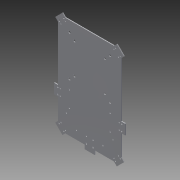
# Autodesk Inventor part: Main Plate
Saved by Autodesk Inventor 2013 (Build 170138000, 138)
## iProperties
Created: 2014-05-12
Part Number: Main Plate
Material: アルミニウム 6061
Document SubType Name: Modeling
Designer: andou
Density: 2.71 g/cm^3
Mass: 218.036 g
Surface Area: 829.556 cm^2
Volume: 80.4562 cm^3
Author: andou
Autodesk Inventor part; units mm, degrees
ref_plane "YZ Plane" through (0, 0, 0) normal (1, 0, 0) x (0, 1, 0)
ref_plane "XZ Plane" through (0, 0, 0) normal (0, 1, 0) x (-1, 0, 0)
ref_plane "XY Plane" through (0, 0, 0) normal (0, 0, 1) x (1, 0, 0)
sketch "スケッチ1" plane through (0, 0, 0) normal (0, 1, 0) x (-1, 0, 0)
  line L0 (-84.7487, 117.8934) -> (-67.0711, 135.5711)
  line L1 (-67.0711, 135.5711) -> (-60, 128.5)
  line L2 (-60, 128.5) -> (0, 128.5)
  line L3 (-84.7487, 117.8934) -> (-77.6777, 110.8223)
  line L4 (-77.6777, 110.8223) -> (-77.6777, -24.1777)
  line L5 (-77.6777, -24.1777) -> (-87.6777, -24.1777)
  line L6 (-87.6777, -24.1777) -> (-87.6777, -49.1777)
  line L7 (-87.6777, -49.1777) -> (-77.6777, -49.1777)
  line L8 (-77.6777, -49.1777) -> (-77.6777, -100.8223)
  line L9 (-77.6777, -100.8223) -> (-84.7487, -107.8934)
  line L10 (-84.7487, -107.8934) -> (-67.0711, -125.5711)
  line L11 (-67.0711, -125.5711) -> (-60, -118.5)
  line L12 (-60, -118.5) -> (-12.5, -118.5)
  line L13 (-12.5, -118.5) -> (-12.5, -128.5)
  line L14 (-12.5, -128.5) -> (0, -128.5)
  line L15 (0, -128.5) -> (0, 128.5)
  line L16 (84.7487, 117.8934) -> (67.0711, 135.5711)
  line L17 (67.0711, 135.5711) -> (60, 128.5)
  line L18 (60, 128.5) -> (0, 128.5)
  line L19 (84.7487, 117.8934) -> (77.6777, 110.8223)
  line L20 (77.6777, 110.8223) -> (77.6777, -24.1777)
  line L21 (77.6777, -24.1777) -> (87.6777, -24.1777)
  line L22 (87.6777, -24.1777) -> (87.6777, -49.1777)
  line L23 (87.6777, -49.1777) -> (77.6777, -49.1777)
  line L24 (77.6777, -49.1777) -> (77.6777, -100.8223)
  line L25 (77.6777, -100.8223) -> (84.7487, -107.8934)
  line L26 (84.7487, -107.8934) -> (67.0711, -125.5711)
  line L27 (67.0711, -125.5711) -> (60, -118.5)
  line L28 (60, -118.5) -> (12.5, -118.5)
  line L29 (12.5, -118.5) -> (12.5, -128.5)
  line L30 (12.5, -128.5) -> (0, -128.5)
  point P0 (0, 0)
  dimension "d0" = 135
  dimension "d2" = 135
  dimension "d4" = 10
  dimension "d6" = 128.5
  dimension "d8" = 25
  dimension "d9" = 257
  dimension "d10" = 12.5
  dimension "d12" = 60
  dimension "d13" = 0
  dimension "d40" = 10
  constraints: 62 end point, 14 symmetric about line, 12 perpendicular, 7 equal length, 2 parallel, 1 horizontal
  measures "d0" distance of L3.end L4.end
  measures "d2" angle of L2 L1
  measures "d4" distance of L0.end L1.end
  measures "d6" distance of L2.end point (0, 0)
  measures "d8" distance of L5.end L6.end
  measures "d9" distance of L14.end L2.end
  measures "d10" distance of L13.end L14.end
  measures "d12" distance of L1.end L2.end
  measures "d13" distance from line of point (0, 0) L15
  measures "d40" distance of L8.end L9.end
extrude "押し出し1" add sketch "スケッチ1" along normal blind 2
sketch "スケッチ2" plane through (0, 2, 0) normal (0, 1, 0) x (1, 0, 0)
  line L0 (12.5, 128.5) -> (-12.5, 128.5) projected
  line L1 (-67.0711, 125.5711) -> (-84.7487, 107.8934) projected
  line L2 (-84.7487, 107.8934) -> (-77.6777, 100.8223) projected
  line L3 (-87.6777, 49.1777) -> (-87.6777, 24.1777) projected
  line L4 (-87.6777, 24.1777) -> (-77.6777, 24.1777) projected
  line L5 (-84.7487, -117.8934) -> (-67.0711, -135.5711) projected
  line L6 (-67.0711, -135.5711) -> (-60, -128.5) projected
  line L7 (-60, -128.5) -> (60, -128.5) projected
  circle A0 centre (-59.6464, 111.7825) radius 1.6
  circle A1 centre (-70.9602, 100.4688) radius 1.6
  circle A2 centre (-8, 98.5) radius 1.6
  circle A3 centre (-72.6777, 44.6777) radius 1.6
  circle A4 centre (-72.6777, 28.6777) radius 1.6
  circle A5 centre (-70.9602, -110.4688) radius 1.6
  circle A6 centre (-59.6464, -121.7825) radius 1.6
  line L8 (0, 128.5) -> (0, -128.5)
  circle A7 centre (59.6464, 111.7825) radius 1.6
  circle A8 centre (70.9602, 100.4688) radius 1.6
  circle A9 centre (8, 98.5) radius 1.6
  circle A10 centre (72.6777, 44.6777) radius 1.6
  circle A11 centre (72.6777, 28.6777) radius 1.6
  circle A12 centre (70.9602, -110.4688) radius 1.6
  circle A13 centre (59.6464, -121.7825) radius 1.6
  point P0 (0, 0)
  dimension "d16" = 3.2
  dimension "d17" = 30
  dimension "d18" = 8
  dimension "d21" = 15
  dimension "d22" = 15
  dimension "d23" = 16
  dimension "d24" = 4.5
  dimension "d25" = 15
  dimension "d26" = 15
  dimension "d27" = 16
  dimension "d28" = 4.5
  dimension "d29" = 15
  dimension "d30" = 15
  dimension "d31" = 16
  dimension "d32" = 4.5
  constraints: 14 centre point, 7 symmetric about line, 6 equal radius, 2 end point, 2 midpoint, 7 other
  measures "d16" diameter of A2
  measures "d17" distance from line of L0 A2.centre
  measures "d18" distance from line of L8 A2.centre
  measures "d21" distance from line of L1 A0.centre
  measures "d22" distance from line of L1 A1.centre
  measures "d23" distance of A0.centre A1.centre
  measures "d24" distance from line of L2 A1.centre
  measures "d25" distance from line of L3 A3.centre
  measures "d26" distance from line of L3 A4.centre
  measures "d27" distance of A3.centre A4.centre
  measures "d28" distance from line of A4.centre L4
  measures "d29" distance from line of A5.centre L5
  measures "d30" distance from line of A6.centre L5
  measures "d31" distance of A5.centre A6.centre
  measures "d32" distance from line of L6 A6.centre
hole "穴1" at (-59.6464, 2, -111.7825) at (-70.9602, 2, -100.4688) at (-72.6777, 2, -44.6777) at (-72.6777, 2, -28.6777) at (-8, 2, -98.5) at (8, 2, -98.5) at (59.6464, 2, -111.7825) at (70.9602, 2, -100.4688) at (-70.9602, 2, 110.4688) at (-59.6464, 2, 121.7825) at (59.6464, 2, 121.7825) at (70.9602, 2, 110.4688) at (72.6777, 2, -28.6777) at (72.6777, 2, -44.6777) direction (0, -1, 0) diameter 3.5 end through all
sketch "スケッチ3" plane through (0, 0, 0) normal (0, -1, 0) x (1, 0, 0)
  line L0 (-60, 128.5) -> (60, 128.5) projected
  circle A0 centre (-37.5, 90) radius 2.5
  circle A1 centre (-50, 102.5) radius 2.5
  circle A2 centre (-37.5, 15) radius 2.5
  circle A3 centre (-50, 2.5) radius 2.5
  line L1 (0, 0) -> (0, 128.5)
  circle A4 centre (37.5, 90) radius 2.5
  circle A5 centre (50, 2.5) radius 2.5
  circle A6 centre (37.5, 90) radius 2.5
  circle A7 centre (50, 102.5) radius 2.5
  circle A8 centre (37.5, 15) radius 2.5
  circle A9 centre (50, 2.5) radius 2.5
  dimension "d41" = 5
  dimension "d44" = 100
  dimension "d45" = 75
  dimension "d46" = 12.5
  dimension "d47" = 37.5
  dimension "d48" = 50
  dimension "d49" = 37.5
  dimension "d50" = 50
  dimension "d51" = 15
  constraints: 10 centre point, 8 symmetric about line, 3 equal radius, 2 end point, 1 midpoint, 6 other
  measures "d41" diameter of A1
  measures "d44" distance of A1.centre A3.centre
  measures "d45" distance of A0.centre A2.centre
  measures "d46" horizontal distance of A1.centre A0.centre
  measures "d47" horizontal distance of A2.centre L1.start
  measures "d48" horizontal distance of L1.start A3.centre
  measures "d49" horizontal distance of L1.start A0.centre
  measures "d50" horizontal distance of L1.start A1.centre
  measures "d51" vertical distance of A2.centre L1.start
hole "穴2" at (-37.5, 0, 90) at (-50, 0, 102.5) at (-37.5, 0, 15) at (-50, 0, 2.5) at (37.5, 0, 15) at (50, 0, 2.5) at (37.5, 0, 90) at (50, 0, 102.5) direction (0, 1, 0) diameter 5.5 end through all
sketch "スケッチ5" plane through (0, 2, 0) normal (0, 1, 0) x (1, 0, 0)
  line L0 (77.6777, 100.8223) -> (84.7487, 107.8934) projected
  line L1 (84.7487, 107.8934) -> (67.0711, 125.5711) projected
  line L2 (-67.0711, 125.5711) -> (-84.7487, 107.8934) projected
  line L3 (-84.7487, 107.8934) -> (-77.6777, 100.8223) projected
  circle A0 centre (-57.1716, 73.2452) radius 1.5
  circle A1 centre (-32.4228, 97.9939) radius 1.5
  circle A2 centre (32.4228, 97.9939) radius 1.5
  circle A3 centre (57.1716, 73.2452) radius 1.5
  line L4 (-32.4228, 97.9939) -> (-57.1716, 73.2452)
  line L5 (32.4228, 97.9939) -> (57.1716, 73.2452)
  circle A4 centre (-75.2028, 104.7114) radius 1.5
  circle A5 centre (-63.8891, 116.0251) radius 1.5
  circle A6 centre (37.5, -90) radius 2.75 projected
  circle A7 centre (37.5, -15) radius 2.75 projected
  circle A8 centre (-37.5, -15) radius 2.75 projected
  circle A9 centre (-37.5, -90) radius 2.75 projected
  circle A10 centre (-50, -102.5) radius 2.75 projected
  circle A11 centre (-50, -2.5) radius 2.75 projected
  circle A12 centre (50, -2.5) radius 2.75 projected
  circle A13 centre (50, -102.5) radius 2.75 projected
  circle A14 centre (72.6777, 28.6777) radius 1.75 projected
  circle A15 centre (59.6464, -121.7825) radius 1.75 projected
  circle A16 centre (-70.9602, -110.4688) radius 1.75 projected
  circle A17 centre (59.6464, 111.7825) radius 1.75 projected
  circle A18 centre (-8, 98.5) radius 1.75 projected
  circle A19 centre (-72.6777, 44.6777) radius 1.75 projected
  circle A20 centre (-59.6464, 111.7825) radius 1.75 projected
  circle A21 centre (-70.9602, 100.4688) radius 1.75 projected
  circle A22 centre (-72.6777, 28.6777) radius 1.75 projected
  circle A23 centre (8, 98.5) radius 1.75 projected
  circle A24 centre (70.9602, 100.4688) radius 1.75 projected
  circle A25 centre (-59.6464, -121.7825) radius 1.75 projected
  circle A26 centre (70.9602, -110.4688) radius 1.75 projected
  circle A27 centre (72.6777, 44.6777) radius 1.75 projected
  line L6 (84.7487, -117.8934) -> (77.6777, -110.8223) projected
  line L7 (77.6777, -110.8223) -> (77.6777, 24.1777) projected
  line L8 (77.6777, 24.1777) -> (87.6777, 24.1777) projected
  line L9 (87.6777, 24.1777) -> (87.6777, 49.1777) projected
  line L10 (87.6777, 49.1777) -> (77.6777, 49.1777) projected
  line L11 (77.6777, 49.1777) -> (77.6777, 100.8223) projected
  line L12 (77.6777, 100.8223) -> (84.7487, 107.8934) projected
  line L13 (84.7487, 107.8934) -> (67.0711, 125.5711) projected
  line L14 (67.0711, 125.5711) -> (60, 118.5) projected
  line L15 (60, 118.5) -> (12.5, 118.5) projected
  line L16 (12.5, 118.5) -> (12.5, 128.5) projected
  line L17 (12.5, 128.5) -> (-12.5, 128.5) projected
  line L18 (-12.5, 128.5) -> (-12.5, 118.5) projected
  line L19 (-12.5, 118.5) -> (-60, 118.5) projected
  line L20 (-60, 118.5) -> (-67.0711, 125.5711) projected
  line L21 (-67.0711, 125.5711) -> (-84.7487, 107.8934) projected
  line L22 (-84.7487, 107.8934) -> (-77.6777, 100.8223) projected
  line L23 (-77.6777, 100.8223) -> (-77.6777, 49.1777) projected
  line L24 (-77.6777, 49.1777) -> (-87.6777, 49.1777) projected
  line L25 (-87.6777, 49.1777) -> (-87.6777, 24.1777) projected
  line L26 (-87.6777, 24.1777) -> (-77.6777, 24.1777) projected
  line L27 (-77.6777, 24.1777) -> (-77.6777, -110.8223) projected
  line L28 (-77.6777, -110.8223) -> (-84.7487, -117.8934) projected
  line L29 (-84.7487, -117.8934) -> (-67.0711, -135.5711) projected
  line L30 (-67.0711, -135.5711) -> (-60, -128.5) projected
  line L31 (-60, -128.5) -> (60, -128.5) projected
  line L32 (60, -128.5) -> (67.0711, -135.5711) projected
  line L33 (67.0711, -135.5711) -> (84.7487, -117.8934) projected
  line L34 (-75.2028, 104.7114) -> (-63.8891, 116.0251)
  circle A28 centre (63.8891, 116.0251) radius 1.5
  circle A29 centre (75.2028, 104.7114) radius 1.5
  line L35 (63.8891, 116.0251) -> (75.2028, 104.7114)
  point P0 (0, 0)
  dimension "d64" = 3
  dimension "d65" = 35
  dimension "d68" = 5
  dimension "d69" = 5
  dimension "d77" = 16
  dimension "d80" = 4.5
  dimension "d82" = 4.5
  dimension "d83" = 16
  dimension "d129" = 6
  dimension "d130" = 35
  dimension "d131" = 6
  dimension "d132" = 35
  constraints: 8 centre point, 8 end point, 7 equal radius, 3 perpendicular, 2 parallel, 1 coincident
  measures "d64" diameter of A1
  measures "d65" distance of A1.centre L4.end
  measures "d68" distance from line of L4.end L3
  measures "d69" distance from line of L0 L5.end
  measures "d77" distance of L34.end L34.start
  measures "d80" distance from line of L3 L34.start
  measures "d82" distance from line of L0 L35.end
  measures "d83" distance of L35.start L35.end
  measures "d129" distance from line of L34 A20.centre
  measures "d130" distance between parallel lines of L4 L34
  measures "d131" distance from line of L35 A24.centre
  measures "d132" distance between parallel lines of L35 L5
hole "穴4" at (-75.2028, 2, -104.7114) at (-63.8891, 2, -116.0251) at (-57.1716, 2, -73.2452) at (-32.4228, 2, -97.9939) at (32.4228, 2, -97.9939) at (57.1716, 2, -73.2452) at (75.2028, 2, -104.7114) at (63.8891, 2, -116.0251) direction (0, -1, 0) diameter 3.5 end through all
sketch "スケッチ6" plane through (0, 2, 0) normal (0, 1, 0) x (1, 0, 0)
  circle A0 centre (-50, 60) radius 1.75
  circle A1 centre (-50, 20) radius 1.75
  circle A2 centre (50, 60) radius 1.75
  circle A3 centre (50, 20) radius 1.75
  point P0 (0, 0)
  dimension "d91" = 100
  dimension "d93" = 100
  dimension "d94" = 40
  dimension "d95" = 40
  dimension "d96" = 3.5
  dimension "d97" = 60
  dimension "d98" = 60
  dimension "d99" = 50
  dimension "d100" = 50
  constraints: 4 centre point, 3 equal radius
  measures "d91" distance of A2.centre A0.centre
  measures "d93" distance of A3.centre A1.centre
  measures "d94" distance of A0.centre A1.centre
  measures "d95" distance of A2.centre A3.centre
  measures "d96" diameter of A2
  measures "d97" vertical distance of point (0, 0) A0.centre
  measures "d98" vertical distance of point (0, 0) A2.centre
  measures "d99" horizontal distance of point (0, 0) A3.centre
  measures "d100" horizontal distance of point (0, 0) A0.centre
hole "穴5" at (-50, 2, -60) at (-50, 2, -20) at (50, 2, -60) at (50, 2, -20) direction (0, -1, 0) diameter 3.5 end through all
sketch "スケッチ7" plane through (0, 2, 0) normal (0, 1, 0) x (1, 0, 0)
  circle A0 centre (50, 60) radius 1.75 projected
  circle A1 centre (-50, 60) radius 1.75 projected
  circle A2 centre (-50, 20) radius 1.75 projected
  circle A3 centre (50, 20) radius 1.75 projected
  circle A4 centre (75.2028, 104.7114) radius 1.75 projected
  circle A5 centre (32.4228, 97.9939) radius 1.75 projected
  circle A6 centre (-57.1716, 73.2452) radius 1.75 projected
  circle A7 centre (-75.2028, 104.7114) radius 1.75 projected
  circle A8 centre (-63.8891, 116.0251) radius 1.75 projected
  circle A9 centre (-32.4228, 97.9939) radius 1.75 projected
  circle A10 centre (57.1716, 73.2452) radius 1.75 projected
  circle A11 centre (63.8891, 116.0251) radius 1.75 projected
  circle A12 centre (37.5, -90) radius 2.75 projected
  circle A13 centre (37.5, -15) radius 2.75 projected
  circle A14 centre (-37.5, -15) radius 2.75 projected
  circle A15 centre (-37.5, -90) radius 2.75 projected
  circle A16 centre (-50, -102.5) radius 2.75 projected
  circle A17 centre (-50, -2.5) radius 2.75 projected
  circle A18 centre (50, -2.5) radius 2.75 projected
  circle A19 centre (50, -102.5) radius 2.75 projected
  circle A20 centre (72.6777, 28.6777) radius 1.75 projected
  circle A21 centre (59.6464, -121.7825) radius 1.75 projected
  circle A22 centre (-70.9602, -110.4688) radius 1.75 projected
  circle A23 centre (59.6464, 111.7825) radius 1.75 projected
  circle A24 centre (-8, 98.5) radius 1.75 projected
  circle A25 centre (-72.6777, 44.6777) radius 1.75 projected
  circle A26 centre (-59.6464, 111.7825) radius 1.75 projected
  circle A27 centre (-70.9602, 100.4688) radius 1.75 projected
  circle A28 centre (-72.6777, 28.6777) radius 1.75 projected
  circle A29 centre (8, 98.5) radius 1.75 projected
  circle A30 centre (70.9602, 100.4688) radius 1.75 projected
  circle A31 centre (-59.6464, -121.7825) radius 1.75 projected
  circle A32 centre (70.9602, -110.4688) radius 1.75 projected
  circle A33 centre (72.6777, 44.6777) radius 1.75 projected
  line L0 (84.7487, -117.8934) -> (77.6777, -110.8223) projected
  line L1 (77.6777, -110.8223) -> (77.6777, 24.1777) projected
  line L2 (77.6777, 24.1777) -> (87.6777, 24.1777) projected
  line L3 (87.6777, 24.1777) -> (87.6777, 49.1777) projected
  line L4 (87.6777, 49.1777) -> (77.6777, 49.1777) projected
  line L5 (77.6777, 49.1777) -> (77.6777, 100.8223) projected
  line L6 (77.6777, 100.8223) -> (84.7487, 107.8934) projected
  line L7 (84.7487, 107.8934) -> (67.0711, 125.5711) projected
  line L8 (67.0711, 125.5711) -> (60, 118.5) projected
  line L9 (60, 118.5) -> (12.5, 118.5) projected
  line L10 (12.5, 118.5) -> (12.5, 128.5) projected
  line L11 (12.5, 128.5) -> (-12.5, 128.5) projected
  line L12 (-12.5, 128.5) -> (-12.5, 118.5) projected
  line L13 (-12.5, 118.5) -> (-60, 118.5) projected
  line L14 (-60, 118.5) -> (-67.0711, 125.5711) projected
  line L15 (-67.0711, 125.5711) -> (-84.7487, 107.8934) projected
  line L16 (-84.7487, 107.8934) -> (-77.6777, 100.8223) projected
  line L17 (-77.6777, 100.8223) -> (-77.6777, 49.1777) projected
  line L18 (-77.6777, 49.1777) -> (-87.6777, 49.1777) projected
  line L19 (-87.6777, 49.1777) -> (-87.6777, 24.1777) projected
  line L20 (-87.6777, 24.1777) -> (-77.6777, 24.1777) projected
  line L21 (-77.6777, 24.1777) -> (-77.6777, -110.8223) projected
  line L22 (-77.6777, -110.8223) -> (-84.7487, -117.8934) projected
  line L23 (-84.7487, -117.8934) -> (-67.0711, -135.5711) projected
  line L24 (-67.0711, -135.5711) -> (-60, -128.5) projected
  line L25 (-60, -128.5) -> (60, -128.5) projected
  line L26 (60, -128.5) -> (67.0711, -135.5711) projected
  line L27 (67.0711, -135.5711) -> (84.7487, -117.8934) projected
  line L28 (-30, 60) -> (0, 47.5736)
  line L29 (0, 47.5736) -> (30, 60)
  line L30 (30, 60) -> (-30, 60)
  line L31 (-50, 50) -> (-50, 30)
  line L32 (-50, 30) -> (-12.6795, 40)
  line L33 (-12.6795, 40) -> (-50, 50)
  line L34 (-38.2518, -17.6489) -> (-36.0663, -17.3467)
  line L35 (-38.2518, -17.6452) -> (-38.2518, -17.6489)
  line L36 (-30, 0) -> (30, 0)
  line L37 (30, 0) -> (0, -30)
  line L38 (0, -30) -> (-30, 0)
  line L39 (0, 60) -> (0, 20)
  line L40 (-50, 40) -> (50, 40)
  line L41 (-50, -2.5) -> (0, -52.5)
  line L42 (50, -2.5) -> (0, -52.5)
  line L43 (-52.5, -82.5) -> (-52.5, -22.5)
  line L44 (-52.5, -22.5) -> (-22.5, -52.5)
  line L45 (-22.5, -52.5) -> (-52.5, -82.5)
  line L46 (30, -105) -> (-30, -105)
  line L47 (-30, -105) -> (0, -75)
  line L48 (0, -75) -> (30, -105)
  line L49 (52.5, -22.5) -> (52.5, -82.5)
  line L50 (52.5, -82.5) -> (22.5, -52.5)
  line L51 (22.5, -52.5) -> (52.5, -22.5)
  line L52 (-30, 20) -> (0, 32.4264)
  line L53 (0, 32.4264) -> (30, 20)
  line L54 (30, 20) -> (-30, 20)
  line L55 (50, 50) -> (50, 30)
  line L56 (50, 30) -> (12.6795, 40)
  line L57 (12.6795, 40) -> (50, 50)
  point P0 (0, 0)
  dimension "d109" = 135
  dimension "d110" = 60
  dimension "d112" = 20
  dimension "d113" = 0
  dimension "d114" = 0
  dimension "d115" = 20
  dimension "d116" = 10
  dimension "d117" = 30
  dimension "d119" = 60
  dimension "d120" = 20
  dimension "d121" = 90
  dimension "d122" = 0
  dimension "d125" = 360
  constraints: 60 end point, 7 perpendicular, 6 symmetric about line, 3 equal length, 2 midpoint, 2 point on circle, 1 parallel, 25 other
  measures "d109" angle of L29 L28
  measures "d110" distance of L29.end L28.start
  measures "d112" distance of A0.centre L29.end
  measures "d113" distance from line of A0.centre L30
  measures "d114" distance from line of A2.centre L31
  measures "d115" distance of L31.start L31.end
  measures "d116" distance of A1.centre L31.start
  measures "d117" angle of L33 L32
  measures "d119" distance of L36.start L36.end
  measures "d120" horizontal distance of L42.start L36.end
  measures "d121" angle of L37 L38
  measures "d122" distance from line of point (0, 0) L36
extrude "押し出し2" [suppressed]
sketch "スケッチ9" plane through (0, 0, 0) normal (0, -1, 0) x (1, 0, 0)
  circle A0 centre (-70.9602, 110.4688) radius 1.75 projected
  circle A1 centre (-8, -98.5) radius 1.75 projected
  circle A2 centre (-72.6777, -44.6777) radius 1.75 projected
  circle A3 centre (-59.6464, 121.7825) radius 1.75 projected
  line L0 (-60, 128.5) -> (60, 128.5) projected
  line L1 (-67.0711, 135.5711) -> (-60, 128.5) projected
  line L2 (-77.6777, 110.8223) -> (-84.7487, 117.8934) projected
  line L3 (-87.6777, -49.1777) -> (-87.6777, -24.1777) projected
  line L4 (-77.6777, -49.1777) -> (-87.6777, -49.1777) projected
  line L5 (-12.5, -128.5) -> (-12.5, -118.5) projected
  line L6 (12.5, -128.5) -> (-12.5, -128.5) projected
  line L7 (77.6777, 110.8223) -> (77.6777, -24.1777) projected
  circle A4 centre (-78.6777, -28.6777) radius 2
  circle A5 centre (-78.6777, -44.6777) radius 2
  circle A6 centre (-63.8891, 126.0251) radius 2
  circle A7 centre (-75.2028, 114.7114) radius 2
  line L8 (-78.6777, -44.6777) -> (-78.6777, -28.6777)
  line L9 (-75.2028, 114.7114) -> (-63.8891, 126.0251)
  line L10 (0, 128.5) -> (0, -128.5)
  circle A8 centre (-8, -114.5) radius 2
  circle A9 centre (78.6777, -28.6777) radius 2
  circle A10 centre (78.6777, -44.6777) radius 2
  circle A11 centre (63.8891, 126.0251) radius 2
  circle A12 centre (75.2028, 114.7114) radius 2
  circle A13 centre (8, -114.5) radius 2
  point P0 (0, 0)
  dimension "d133" = 4
  dimension "d135" = 6
  dimension "d136" = 4.5
  dimension "d137" = 16
  dimension "d142" = 4.5
  dimension "d143" = 4.5
  dimension "d144" = 6
  dimension "d145" = 6
  dimension "d146" = 16
  dimension "d147" = 4.5
  constraints: 10 centre point, 6 end point, 5 symmetric about line, 4 equal radius, 2 midpoint, 2 parallel, 5 other
  measures "d133" diameter of A6
  measures "d135" distance from line of A2.centre L8
  measures "d136" distance from line of L4 L8.start
  measures "d137" distance of L8.start L8.end
  measures "d142" distance from line of L9.start L2
  measures "d143" distance from line of L1 L9.end
  measures "d144" distance of L9.end A3.centre
  measures "d145" distance of L9.start A0.centre
  measures "d146" distance of A1.centre A8.centre
  measures "d147" distance from line of L5 A8.centre
hole "穴6" at (78.6777, 0, -28.6777) at (78.6777, 0, -44.6777) at (8, 0, -114.5) at (-8, 0, -114.5) at (-78.6777, 0, -44.6777) at (-78.6777, 0, -28.6777) at (-75.2028, 0, 114.7114) at (-63.8891, 0, 126.0251) at (63.8891, 0, 126.0251) at (75.2028, 0, 114.7114) direction (0, 1, 0) diameter 4 end through all
